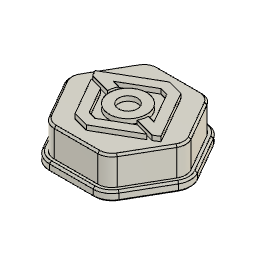
LDO Bestagon Insert (Autodesk Fusion 360 design; units mm, degrees)
Autodesk Fusion 360 part; units mm, degrees
sketch "Sketch1" plane through (0, 0, 0) normal (0, 0, 1) x (1, 0, 0)
  line L0 (-6.3509, 11) -> (-12.7017, 0)
  line L1 (-12.7017, 0) -> (-6.3509, -11)
  line L2 (-6.3509, -11) -> (6.3509, -11)
  line L3 (6.3509, -11) -> (12.7017, 0)
  line L4 (12.7017, 0) -> (6.3509, 11)
  line L5 (6.3509, 11) -> (-6.3509, 11)
  dimension "d1" = 11
  measures "d1" distance of origin L5
extrude "Extrude1" add sketch "Sketch1" along normal blind 6
fillet "Fillet1" radius 3 6 edges at (6.3509, -11, 3) (12.7017, 0, 3) (-6.3509, -11, 3) (-12.7017, 0, 3) (-6.3509, 11, 3) (6.3509, 11, 3)
sketch "Sketch2" plane through (0, 0, 0) normal (0, 0, -1) x (1, 0, 0)
  arc A0 (4.6188, -11) -> (7.2169, -9.5) centre (4.6188, -8) ccw
  line L0 (7.2169, -9.5) -> (11.8357, -1.5)
  arc A1 (11.8357, -1.5) -> (11.8357, 1.5) centre (9.2376, 0) ccw
  line L1 (11.8357, 1.5) -> (7.2169, 9.5) construction
  arc A2 (7.2169, 9.5) -> (4.6188, 11) centre (4.6188, 8) ccw
  line L2 (4.6188, 11) -> (-4.6188, 11)
  arc A3 (-4.6188, 11) -> (-7.2169, 9.5) centre (-4.6188, 8) ccw
  line L3 (-7.2169, 9.5) -> (-11.8357, 1.5)
  arc A4 (-11.8357, 1.5) -> (-11.8357, -1.5) centre (-9.2376, 0) ccw
  line L4 (-11.8357, -1.5) -> (-7.2169, -9.5)
  arc A5 (-7.2169, -9.5) -> (-4.6188, -11) centre (-4.6188, -8) ccw
  line L5 (-4.6188, -11) -> (4.6188, -11)
  line L6 (-8.0829, 10) -> (-12.7017, 2)
  arc A6 (-12.7017, 2) -> (-12.7017, -2) centre (-9.2376, 0) ccw
  line L7 (-12.7017, -2) -> (-8.0829, -10)
  arc A7 (-8.0829, -10) -> (-4.6188, -12) centre (-4.6188, -8) ccw
  line L8 (-4.6188, -12) -> (4.6188, -12)
  arc A8 (4.6188, -12) -> (8.0829, -10) centre (4.6188, -8) ccw
  line L9 (8.0829, -10) -> (12.7017, -2)
  arc A9 (12.7017, -2) -> (12.7017, 2) centre (9.2376, 0) ccw
  line L10 (12.7017, 2) -> (8.0829, 10)
  arc A10 (8.0829, 10) -> (4.6188, 12) centre (4.6188, 8) ccw
  line L11 (4.6188, 12) -> (-4.6188, 12)
  arc A11 (-4.6188, 12) -> (-8.0829, 10) centre (-4.6188, 8) ccw
  dimension "d6" = 1
extrude "Extrude2" add sketch "Sketch2" along normal blind 2
sketch "Sketch3" plane through (0, 0, 6) normal (0, 0, 1) x (-1, 0, 0)
  arc A0 (-7.2169, -9.5) -> (-4.6188, -11) centre (-4.6188, -8) ccw
  line L0 (-4.6188, -11) -> (4.6188, -11)
  arc A1 (4.6188, -11) -> (7.2169, -9.5) centre (4.6188, -8) ccw
  line L1 (7.2169, -9.5) -> (11.8357, -1.5) construction
  arc A2 (11.8357, -1.5) -> (11.8357, 1.5) centre (9.2376, 0) ccw
  line L2 (11.8357, 1.5) -> (7.2169, 9.5)
  arc A3 (7.2169, 9.5) -> (4.6188, 11) centre (4.6188, 8) ccw
  line L3 (4.6188, 11) -> (-4.6188, 11)
  arc A4 (-4.6188, 11) -> (-7.2169, 9.5) centre (-4.6188, 8) ccw
  line L4 (-7.2169, 9.5) -> (-11.8357, 1.5)
  arc A5 (-11.8357, 1.5) -> (-11.8357, -1.5) centre (-9.2376, 0) ccw
  line L5 (-11.8357, -1.5) -> (-7.2169, -9.5)
  line L6 (8.425, -0.6467) -> (5.7257, 0.0765)
  line L7 (5.6158, -2.5276) -> (4.0271, -2.1019)
  line L8 (5.7257, 0.0765) -> (2.4486, 5.7527)
  line L9 (-4.0271, 2.1019) -> (-8.3151, 3.2509)
  line L10 (-0.4766, -8.3268) -> (9.5251, -2.5523)
  line L11 (-9.5251, 2.5523) -> (-3.7506, -7.4495)
  line L12 (8.425, -0.6467) -> (3.7506, 7.4495)
  line L13 (-0.7558, -6.2062) -> (5.6158, -2.5276)
  line L14 (-4.9203, 2.9291) -> (-7.6196, 3.6524)
  line L15 (-8.3151, 3.2509) -> (-9.5251, 2.5523)
  line L16 (0.7558, 6.2062) -> (-4.9203, 2.9291)
  line L17 (0.4766, 8.3268) -> (-7.6196, 3.6524)
  line L18 (9.5251, -2.5523) -> (8.8265, -1.3422)
  line L19 (-6.1272, 0.6189) -> (-2.4486, -5.7527)
  line L20 (8.8265, -1.3422) -> (4.5385, -0.1932)
  line L21 (3.7506, 7.4495) -> (0.4766, 8.3268)
  line L22 (2.4486, 5.7527) -> (0.7558, 6.2062)
  line L23 (-0.7558, -6.2062) -> (-2.4486, -5.7527)
  line L24 (-0.4766, -8.3268) -> (-3.7506, -7.4495)
  circle A6 centre (0, 0) radius 1.9987
  circle A7 centre (0, 0) radius 3.9748
  arc A8 (-4.0271, 2.1019) -> (-4.5385, 0.1932) centre (0, 0) ccw
  line L25 (-4.5385, 0.1932) -> (-6.1272, 0.6189)
  arc A9 (4.0271, -2.1019) -> (4.5385, -0.1932) centre (0, 0) ccw
extrude "Extrude3" add sketch "Sketch3" along normal blind 1
chamfer "Chamfer1" distance 0.4 angle 45 36 edges at (9.5263, -5.5, 6) (12.2376, 0, 6) (9.5263, 5.5, 6) (6.1188, 10.5981, 6) (0, 11, 6) (-6.1188, 10.5981, 6) (-9.5263, 5.5, 6) (-12.2376, 0, 6) (-9.5263, -5.5, 6) (-6.1188, -10.5981, 6) (0, -11, 6) (6.1188, -10.5981, 6) (10.3923, -6, 0) (6.6188, -11.4641, 0) (0, -12, 0) (-6.6188, -11.4641, 0) (-10.3923, -6, 0) (-13.2376, 0, 0) (-10.3923, 6, 0) (-6.6188, 11.4641, 0) (0, 12, 0) (6.6188, 11.4641, 0) (10.3923, 6, 0) (13.2376, 0, 0) (10.3923, -6, -2) (6.6188, -11.4641, -2) (0, -12, -2) (-6.6188, -11.4641, -2) (-10.3923, -6, -2) (-13.2376, 0, -2) (-10.3923, 6, -2) (-6.6188, 11.4641, -2) (0, 12, -2) (6.6188, 11.4641, -2) (10.3923, 6, -2) (13.2376, 0, -2)
sketch "Sketch4" plane through (0, 0, -2) normal (0, 0, -1) x (1, 0, 0)
  line L0 (12.3553, 1.8) -> (7.7365, 9.8)
  arc A0 (7.7365, 9.8) -> (4.6188, 11.6) centre (4.6188, 8) ccw
  line L1 (4.6188, 11.6) -> (-4.6188, 11.6)
  arc A1 (-4.6188, 11.6) -> (-7.7365, 9.8) centre (-4.6188, 8) ccw
  line L2 (-7.7365, 9.8) -> (-12.3553, 1.8)
  arc A2 (-12.3553, 1.8) -> (-12.3553, -1.8) centre (-9.2376, 0) ccw
  line L3 (-12.3553, -1.8) -> (-7.7365, -9.8)
  arc A3 (-7.7365, -9.8) -> (-4.6188, -11.6) centre (-4.6188, -8) ccw
  line L4 (-4.6188, -11.6) -> (4.6188, -11.6)
  arc A4 (4.6188, -11.6) -> (7.7365, -9.8) centre (4.6188, -8) ccw
  line L5 (7.7365, -9.8) -> (12.3553, -1.8)
  arc A5 (12.3553, -1.8) -> (12.3553, 1.8) centre (9.2376, 0) ccw
  line L6 (0, 0) -> (-6.4188, -11.1177) construction
  line L7 (-3.2094, -5.5588) -> (1.5717, -4.2778)
  line L8 (1.5717, -4.2778) -> (-0.1604, -3.2778)
  line L9 (-0.1604, -3.2778) -> (2.8396, 1.9184)
  line L10 (2.8396, 1.9184) -> (1.5406, 2.6684)
  line L11 (1.5406, 2.6684) -> (0, 0) construction
  line L12 (-3.2094, -5.5588) -> (-4.4905, -0.7778)
  line L13 (-4.4905, -0.7778) -> (-2.7584, -1.7778)
  line L14 (0.2416, 3.4184) -> (1.5406, 2.6684)
  line L15 (-2.7584, -1.7778) -> (0.2416, 3.4184)
  dimension "d14" = 1.5
  dimension "d15" = 2
  dimension "d16" = 45
  dimension "d17" = 6
  constraint coincident L6.start L11.end
  constraint midpoint A3 L6.end
  constraint midpoint L6 L7.start
  constraint perpendicular L6 L8
  constraint perpendicular L8 L9
  constraint perpendicular L9 L10
  constraint perpendicular L10 L11
  constraint symmetric L6 L7.start L12.start
  constraint symmetric L6 L7.end L12.end
  constraint symmetric L6 L8.end L13.end
  constraint symmetric L6 L9.end L14.start
  constraint symmetric L6 L10.end L11.start
  measures "d14" distance of L9.end L10.end
  measures "d15" distance of L7.end L8.end
  measures "d16" angle of L6 L7
  measures "d17" distance of L8.end L9.end
extrude "Extrude4" cut sketch "Sketch4" against normal blind 0.4 contours L7 L8 L9 L10 L12 L13 L14 L15
